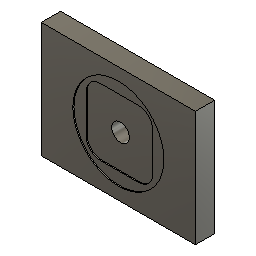
Elara Test v2 (Autodesk Fusion 360 design; units mm, degrees)
Autodesk Fusion 360 part; units mm, degrees
sketch "Sketch1" plane through (0, 0, 0) normal (0, 0, 1) x (1, 0, 0)
  line L0 (0, 0) -> (50.8, 0)
  line L1 (50.8, 0) -> (50.8, 38.1)
  line L2 (50.8, 38.1) -> (0, 38.1)
  line L3 (0, 38.1) -> (0, 0)
  line L4 (0, 19.05) -> (50.8, 19.05) construction
  line L5 (25.4, 38.1) -> (25.4, 0) construction
  circle A0 centre (25.4, 19.05) radius 15
  line L6 (19.1625, 30.05) -> (31.6375, 30.05)
  line L7 (36.4, 25.2875) -> (36.4, 12.8125)
  line L8 (31.6375, 8.05) -> (19.1625, 8.05)
  line L9 (14.4, 12.8125) -> (14.4, 25.2875)
  circle A1 centre (25.4, 19.05) radius 2.9114
  arc A2 (31.6375, 8.05) -> (36.4, 12.8125) centre (31.6375, 12.8125) ccw
  arc A3 (14.4, 12.8125) -> (19.1625, 8.05) centre (19.1625, 12.8125) ccw
  arc A4 (19.1625, 30.05) -> (14.4, 25.2875) centre (19.1625, 25.2875) ccw
  arc A5 (36.4, 25.2875) -> (31.6375, 30.05) centre (31.6375, 25.2875) ccw
  dimension "d1" = 50.8
  dimension "d2" = 38.1
  dimension "d13" = 4.7625
  dimension "d14" = 30
  dimension "d15" = 11
  dimension "d16" = 11
  dimension "d17" = 11
  dimension "d18" = 11
  constraint horizontal L0
  constraint vertical L1
  constraint horizontal L2
  constraint vertical L3
  constraint coincident L0.start L3.end
  constraint midpoint L3 L4.start
  constraint midpoint L1 L4.end
  constraint midpoint L2 L5.start
  constraint midpoint L0 L5.end
  constraint midpoint L5 A0.centre
  constraint horizontal L6
  constraint vertical L7
  constraint horizontal L8
  constraint vertical L9
  constraint concentric A0 A1
  constraint tangent L7 A2
  constraint tangent L8 A2
  constraint tangent L8 A3
  constraint tangent L9 A3
  constraint equal A2 A3
  constraint tangent L6 A4
  constraint tangent L9 A4
  constraint equal A2 A4
  constraint tangent L6 A5
  constraint tangent L7 A5
  constraint equal A2 A5
  measures "d1" distance of L0.start L0.end
  measures "d2" distance of L0.start L2.end
  measures "d13" radius of A2
  measures "d14" diameter of A0
  measures "d15" distance of L5 L7
  measures "d16" distance of L5 L9
  measures "d17" distance of L4 L6
  measures "d18" distance of L4 L8
extrude "Extrude1" add sketch "Sketch1" along normal blind 6.35 contours L0 L1 L2 L3 | A0 | L6 L7 L8 L9 A2 A3 A4 A5 | A1
extrude "Extrude2" cut sketch "Sketch1" against normal blind 0.35 from surface at 6.35 contours A0 | L6 L7 L8 L9 A2 A3 A4 A5 | A1
extrude "Extrude3" cut sketch "Sketch1" against normal blind 0.35 from surface at 6 contours L6 L7 L8 L9 A2 A3 A4 A5 | A1
extrude "Extrude4" cut sketch "Sketch1" against normal through all from surface at 5.65 contours A1
equation "d13 = 0.125 * 1.5 in"
